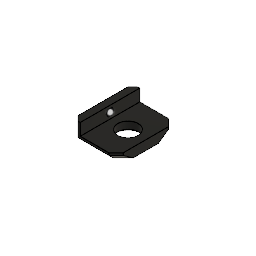
Bed Corner 3P Support (Autodesk Fusion 360 design; units mm, degrees)
Autodesk Fusion 360 part; units mm, degrees
sketch "Sketch3" plane through (-5, 0, 0) normal (1, 0, 0) x (0, 1, 0)
  line L0 (7, 36) -> (57, 36)
  line L1 (57, 36) -> (57, 46)
  line L2 (57, 46) -> (7, 46)
  line L3 (7, 46) -> (57, 36) construction
  line L4 (33.5877, 38.25) -> (35.1754, 41)
  line L5 (35.1754, 41) -> (33.5877, 43.75)
  line L6 (33.5877, 43.75) -> (30.4123, 43.75)
  line L7 (30.4123, 43.75) -> (28.8246, 41)
  line L8 (28.8246, 41) -> (30.4123, 38.25)
  line L9 (30.4123, 38.25) -> (33.5877, 38.25)
  line L10 (7, 46) -> (7, 36)
  point P0 (32, 41)
  dimension "d1" = 5.5
  constraint coincident L2.end L3.start
  constraint coincident L0.end L1.start
  constraint midpoint L3 P0
  constraint horizontal L9
  measures "d1" distance of L6 L9
sketch "Sketch1" plane through (0, 0, 28) normal (0, 0, 1) x (-1, 0, 0)
  line L0 (5, -57) -> (-25, -57)
  line L1 (-25, -57) -> (-25, -7)
  line L2 (-25, -7) -> (5, -7)
  line L3 (5, -7) -> (5, -57)
  line L4 (-25, -7) -> (5, -57) construction
  line L5 (5, -57) -> (11, -57)
  line L6 (11, -57) -> (11, -1)
  line L7 (11, -1) -> (-25, -1)
  line L8 (-25, -1) -> (-25, -7)
  circle A0 centre (-10, -32) radius 2.75
  circle A1 centre (-10, -32) radius 8
  line L9 (5, -7) -> (11, -7)
  dimension "d750" = 30
  dimension "d751" = 50
  dimension "d758" = 6
  dimension "d759" = 6
  dimension "d805" = 0
  dimension "d806" = 0
  dimension "d807" = 0
  dimension "d808" = 0
  dimension "d905" = 0
  dimension "d906" = 0
  dimension "d907" = 0
  dimension "d908" = 0
  dimension "d917" = 0
  dimension "d918" = 0
  dimension "d919" = 0
  dimension "d920" = 0
  dimension "d988" = 0
  dimension "d989" = 0
  dimension "d990" = 0
  dimension "d991" = 0
  dimension "d1049" = 0
  dimension "d1050" = 0
  dimension "d1051" = 0
  dimension "d1052" = 0
  dimension "d1061" = 0
  dimension "d1062" = 0
  dimension "d1063" = 0
  dimension "d1064" = 0
  dimension "d1071" = 0
  dimension "d1072" = 0
  dimension "d1073" = 0
  dimension "d1074" = 0
  dimension "d1243" = 0
  dimension "d1244" = 0
  dimension "d1245" = 0
  dimension "d1246" = 0
  dimension "d1299" = 0
  dimension "d1300" = 0
  dimension "d1301" = 0
  dimension "d1302" = 0
  dimension "d1319" = 0
  dimension "d1320" = 0
  dimension "d1321" = 0
  dimension "d1322" = 0
  constraint horizontal L0
  constraint vertical L1
  constraint horizontal L2
  constraint vertical L3
  constraint perpendicular L3 L5
  constraint perpendicular L5 L6
  constraint perpendicular L1 L7
  constraint perpendicular L2 L8
  constraint midpoint L4 A0.centre
  constraint coincident L6 L9.end
  constraint perpendicular L6 L9
  measures "d750" distance of L0.start L0.end
  measures "d751" distance of L0.start L2.end
  measures "d758" distance of L1.end L7.end
  measures "d759" distance of L0.start L5.end
extrude "Extrude1" add sketch "Sketch1" along normal blind 8 contours L0 L1 L2 L3 | L3 L5 L6 L9
chamfer "Chamfer3" distance 2 angle 45 1 edges at (17.4586, 29.1071, 28)
move_face "OffsetFaces1" offset -0.5 1 faces at (2.0398, 32.7965, 32)
extrude "Extrude2" add sketch "Sketch1" along normal blind 18 contours L3 L5 L6 L9
extrude "Extrude5" cut sketch "Sketch3" against normal blind 3 contours L4 L5 L6 L7 L8 L9
hole "Hole6" at (-5, 32, 41) direction (-1, 0, 0) diameter 3.5 depth 10 tip angle 118
chamfer "Chamfer2" distance 4 angle 45 2 edges at (-11, 57, 37) (-11, 7, 37)
chamfer "Chamfer4" distance 6 angle 45 2 edges at (25, 57, 32) (25, 7, 32)
chamfer "Chamfer1" distance 6 angle 45 7 edges at (-11, 32, 28) (-9, 55, 28) (-9, 9, 28) (6, 7, 28) (6, 57, 28) (22, 54, 28) (22, 10, 28)
equation "d759 = d758"
named bodies: "Bed Corner Support"
